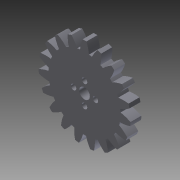
# Autodesk Inventor part: Spur Gear1
Saved by Autodesk Inventor 2013 (Build 170138000, 138)
## iProperties
Created: 2013-02-22
Part Number: Spur Gear1
Material: Steel
Document SubType Name: Modeling
Designer: Nano
Categories: <?xml version="1.0" encoding="UTF-16"?> <MemberInstance><Categories><FamilyTemplate><FamilyTemplateParameter ValueType="xs:double" Id="1" ObjectReferenceKey="da_z" ObjectType="kUserParameterObject"/><FamilyTemplateParameter ValueType="xs:double" Id="2" ObjectReferenceKey="da_b" ObjectType="kUserParameterObject"/><FamilyTemplateParameter ValueType="xs:double" Id="3" ObjectReferenceKey="da_beta" ObjectType="kUserParameterObject"/><FamilyTemplateParameter ValueType="xs:double" Id="4" ObjectReferenceKey="da_da" ObjectType="kUserParameterObject"/><FamilyTemplateParameter ValueType="xs:double" Id="5" ObjectReferenceKey="da_aw" ObjectType="kUserParameterObject"/><FamilyTemplateParameter ValueType="xs:string" Id="6" ObjectReferenceKey="EAIAABAAAAC/AAAAAAAAAIAAAAAAAAAA" ObjectType="83910656" SubObjectId="SurfaceGeometry"/></FamilyTemplate><ParamToTemplateMap><ParamToTemplate CategoryParameter="//CategoryParameter[@InternalName='046C89C9-8512-4d59-83FE-43B91F4F132A']" TemplateParameter="1"/><ParamToTemplate CategoryParameter="//CategoryParameter[@InternalName='2552DF32-E462-4b46-AEBF-C6C7768E72AC']" TemplateParameter="2"/><ParamToTemplate CategoryParameter="//CategoryParameter[@InternalName='C9EE641D-15FC-4fae-A226-E94C4372FDD7']" TemplateParameter="3"/><ParamToTemplate><ParamToTemplate CategoryParameter="//CategoryParameter[@InternalName='00B6519A-459B-49c7-AD84-2E56D39A5744']" ConstantValue="0.000000"/></ParamToTemplate><ParamToTemplate><ParamToTemplate CategoryParameter="//CategoryParameter[@InternalName='04B31F0E-C7A6-4894-AA32-9629BEFACF47']" ConstantValue="1.000000"/></ParamToTemplate><ParamToTemplate><ParamToTemplate CategoryParameter="//CategoryParameter[@InternalName='43CBEC2E-7847-49e7-A936-2F7889FCB2D9']" ConstantValue="0.250000"/></ParamToTemplate><ParamToTemplate><ParamToTemplate CategoryParameter="//CategoryParameter[@InternalName='B1EFC894-105D-4ebd-86BF-FA20ED196853']" ConstantValue="0.350000"/></ParamToTemplate><ParamToTemplate><ParamToTemplate CategoryParameter="//CategoryParameter[@InternalName='51175063-3D10-4879-93E8-6246FE8B403D']" ConstantValue="2060110000.000000"/></ParamToTemplate><ParamToTemplate><ParamToTemplate CategoryParameter="//CategoryParameter[@InternalName='A3A52E27-4454-46a9-B0BD-C932399B70AF']" ConstantValue="0.300000"/></ParamToTemplate><ParamToTemplate><ParamToTemplate CategoryParameter="//CategoryParameter[@InternalName='91B76062-C214-41d9-B1B9-14D2AB99603D']" ConstantValue="0.254000"/></ParamToTemplate><ParamToTemplate><ParamToTemplate CategoryParameter="//CategoryParameter[@InternalName='374E806E-8B8A-4dda-A9AA-1039D6500AD2']" ConstantValue="3.937008"/></ParamToTemplate><ParamToTemplate><ParamToTemplate CategoryParameter="//CategoryParameter[@InternalName='2D373A89-B862-43d6-8D0B-0CBF12AB9F6C']" ConstantValue="0.349066"/></ParamToTemplate><ParamToTemplate CategoryParameter="//CategoryParameter[@InternalName='37777632-D6A2-4fac-9D53-DB8ACD95C989']" TemplateParameter="4"/><ParamToTemplate CategoryParameter="//CategoryParameter[@InternalName='FD1017F1-B727-4f7e-9707-0F86F1FF9423']" TemplateParameter="5"/><ParamToTemplate><ParamToTemplate CategoryParameter="//CategoryParameter[@InternalName='9E1B4470-B2D3-4ff1-B813-535BB4CDF51A']" ConstantValue="3520790.000000"/></ParamToTemplate><ParamToTemplate><ParamToTemplate CategoryParameter="//CategoryParameter[@InternalName='F8452263-BFF6-458c-9FB1-07C4B99E95CD']" ConstantValue="11389170.000000"/></ParamToTemplate><ParamToTemplate><ParamToTemplate CategoryParameter="//CategoryParameter[@InternalName='3E3BB259-FD49-497f-8171-6EBC954A3479']" ConstantValue="2.000000"/></ParamToTemplate><ParamToTemplate CategoryParameter="//CategoryParameter[@InternalName='27C3BAF2-7550-4e4b-AE2C-0DB134B7D9B7']" TemplateParameter="6"/></ParamToTemplateMap><Category DisplayName="Gear" InternalName="DC85795E-93AB-48d5-8EEE-5A27447B64BD" Mnemonic="Gear"><CategoryParameter DisplayName="z" InternalName="046C89C9-8512-4d59-83FE-43B91F4F132A" Mnemonic="z"/><CategoryParameter DisplayName="b" InternalName="2552DF32-E462-4b46-AEBF-C6C7768E72AC" Mnemonic="b"/><CategoryParameter DisplayName="||b|" InternalName="C9EE641D-15FC-4fae-A226-E94C4372FDD7" Mnemonic="beta"/><CategoryParameter DisplayName="x" InternalName="00B6519A-459B-49c7-AD84-2E56D39A5744" Mnemonic="x"/><CategoryParameter DisplayName="a*" InternalName="04B31F0E-C7A6-4894-AA32-9629BEFACF47" Mnemonic="a"/><CategoryParameter DisplayName="c*" InternalName="43CBEC2E-7847-49e7-A936-2F7889FCB2D9" Mnemonic="c"/><CategoryParameter DisplayName="r|.f|*" InternalName="B1EFC894-105D-4ebd-86BF-FA20ED196853" Mnemonic="rf"/><CategoryParameter DisplayName="E" InternalName="51175063-3D10-4879-93E8-6246FE8B403D" Mnemonic="E"/><CategoryParameter DisplayName="||m|" InternalName="A3A52E27-4454-46a9-B0BD-C932399B70AF" Mnemonic="mi"/><Category DisplayName="SpurGear" InternalName="26C5A22E-A91E-4dfd-A3B3-23CCAFAE1764" Mnemonic="SpurGear"><CategoryParameter DisplayName="m" InternalName="91B76062-C214-41d9-B1B9-14D2AB99603D" Mnemonic="m"/><CategoryParameter DisplayName="P" InternalName="374E806E-8B8A-4dda-A9AA-1039D6500AD2" Mnemonic="PP"/><CategoryParameter DisplayName="||a|" InternalName="2D373A89-B862-43d6-8D0B-0CBF12AB9F6C" Mnemonic="alpha"/><CategoryParameter DisplayName="d|.a|" InternalName="37777632-D6A2-4fac-9D53-DB8ACD95C989" Mnemonic="da"/><CategoryParameter DisplayName="a|.w|" InternalName="FD1017F1-B727-4f7e-9707-0F86F1FF9423" Mnemonic="aw"/><CategoryParameter DisplayName="||s||.Flim|" InternalName="9E1B4470-B2D3-4ff1-B813-535BB4CDF51A" Mnemonic="sFlim"/><CategoryParameter DisplayName="||s||.Hlim|" InternalName="F8452263-BFF6-458c-9FB1-07C4B99E95CD" Mnemonic="sHlim"/><CategoryParameter DisplayName="type" InternalName="3E3BB259-FD49-497f-8171-6EBC954A3479" Mnemonic="type"/><CategoryParameter DisplayName="PitchDiameter" InternalName="27C3BAF2-7550-4e4b-AE2C-0DB134B7D9B7" Mnemonic="IDS_PITCHDIAM"/></Category></Category></Categories></MemberInstance>
Density: 1 g/cm^3
CustomPartVersion: 1
Author: Nano
Autodesk Inventor part; units mm, degrees
sketch "Sketch1" plane through (0, 0, 0) normal (0, 0, 1) x (1, 0, 0)
  circle A0 centre (0, 0) radius 26.67
  dimension "d0" = 53.34
  constraints: 1 centre point
  measures "d0" diameter of A0
extrude "Extrusion1" add sketch "Sketch1" along normal blind 6.35
sketch "Sketch2" plane through (0, 0, 0) normal (0, 0, -1) x (-1, 0, 0)
  circle A0 centre (0, 0) radius 26.67 projected
  circle A1 centre (0, 0) radius 24.13
  dimension "d3" = 48.26
  constraints: 1 centre point, 1 coincident
  measures "d3" diameter of A1
surface extrude "Pitch Diameter" sketch "Sketch2" against normal through all shown no curves A1
ref_plane "Work Plane1" through (0, 0, 0) normal (1, 0, 0) x (0, 1, 0)
ref_plane "Work Plane2" through (0, 0, 0) normal (0.9863613, 0.1645946, 0) x (0, 0, 1)
ref_plane "Work Plane3" through (0, 0, 3.175) normal (0, 0, -1) x (-1, 0, 0)
spur gear teeth "Spur Gear" teeth 19 pitch diameter 48.26 tip diameter 53.34 root diameter 41.91 face width 6.35 start plane through (0, 0, 0) normal (0, 0, -1) x (-1, 0, 0)
sketch "Sketch3" plane through (0, 0, 6.35) normal (0, 0, 1) x (1, 0, 0)
  arc A0 (-9.6948, 24.8455) -> (-9.2034, 18.8258) centre (10.7599, 23.4853) ccw projected
  arc A1 (-9.2034, 18.8258) -> (-10.7266, 18.0015) centre (0, 0) ccw projected
  arc A2 (-10.7266, 18.0015) -> (-15.4973, 21.7053) centre (-25.5462, 3.8374) ccw projected
  arc A3 (-15.4973, 21.7053) -> (-17.2368, 20.3515) centre (0, 0) ccw projected
  arc A4 (-17.2368, 20.3515) -> (-14.8174, 14.8174) centre (2.5512, 25.7066) ccw projected
  arc A5 (-14.8174, 14.8174) -> (-15.9904, 13.5432) centre (0, 0) ccw projected
  arc A6 (-15.9904, 13.5432) -> (-21.7053, 15.4973) centre (-25.4081, -4.6654) ccw projected
  arc A7 (-21.7053, 15.4973) -> (-22.911, 13.652) centre (0, 0) ccw projected
  arc A8 (-22.911, 13.652) -> (-18.8258, 9.2034) centre (-5.9339, 25.1421) ccw projected
  arc A9 (-18.8258, 9.2034) -> (-19.5215, 7.6173) centre (0, 0) ccw projected
  arc A10 (-19.5215, 7.6173) -> (-25.5613, 7.6099) centre (-22.5166, -12.6626) ccw projected
  arc A11 (-25.5613, 7.6099) -> (-26.1024, 5.4731) centre (0, 0) ccw projected
  arc A12 (-26.1024, 5.4731) -> (-20.7941, 2.592) centre (-13.776, 21.8531) ccw projected
  arc A13 (-20.7941, 2.592) -> (-20.9371, 0.866) centre (0, 0) ccw projected
  arc A14 (-20.9371, 0.866) -> (-26.6472, -1.1021) centre (-17.185, -19.2876) ccw projected
  arc A15 (-26.6472, -1.1021) -> (-26.4652, -3.2989) centre (0, 0) ccw projected
  arc A16 (-26.4652, -3.2989) -> (-20.509, -4.3003) centre (-20.1253, 16.196) ccw projected
  arc A17 (-20.509, -4.3003) -> (-20.0838, -5.9792) centre (0, 0) ccw projected
  arc A18 (-20.0838, -5.9792) -> (-24.8455, -9.6948) centre (-9.9912, -23.8225) ccw projected
  arc A19 (-24.8455, -9.6948) -> (-23.9601, -11.7134) centre (0, 0) ccw projected
  arc A20 (-23.9601, -11.7134) -> (-18.0015, -10.7266) centre (-24.2937, 8.7838) ccw projected
  arc A21 (-18.0015, -10.7266) -> (-17.0542, -12.1765) centre (0, 0) ccw projected
  arc A22 (-17.0542, -12.1765) -> (-20.3515, -17.2368) centre (-1.7147, -25.7759) ccw projected
  arc A23 (-20.3515, -17.2368) -> (-18.8585, -18.8585) centre (0, 0) ccw projected
  arc A24 (-18.8585, -18.8585) -> (-13.5432, -15.9904) centre (-25.8294, 0.4197) ccw projected
  arc A25 (-13.5432, -15.9904) -> (-12.1765, -17.0542) centre (0, 0) ccw projected
  arc A26 (-12.1765, -17.0542) -> (-13.652, -22.911) centre (6.7476, -24.936) ccw projected
  arc A27 (-13.652, -22.911) -> (-11.7134, -23.9601) centre (0, 0) ccw projected
  arc A28 (-11.7134, -23.9601) -> (-7.6173, -19.5215) centre (-24.5662, -7.9898) ccw projected
  arc A29 (-7.6173, -19.5215) -> (-5.9792, -20.0838) centre (0, 0) ccw projected
  arc A30 (-5.9792, -20.0838) -> (-5.4731, -26.1024) centre (14.4787, -21.394) ccw projected
  arc A31 (-5.4731, -26.1024) -> (-3.2989, -26.4652) centre (0, 0) ccw projected
  arc A32 (-3.2989, -26.4652) -> (-0.866, -20.9371) centre (-20.6408, -15.5336) ccw projected
  arc A33 (-0.866, -20.9371) -> (0.866, -20.9371) centre (0, 0) ccw projected
  arc A34 (0.866, -20.9371) -> (3.2989, -26.4652) centre (20.6408, -15.5336) ccw projected
  arc A35 (3.2989, -26.4652) -> (5.4731, -26.1024) centre (0, 0) ccw projected
  arc A36 (5.4731, -26.1024) -> (5.9792, -20.0838) centre (-14.4787, -21.394) ccw projected
  arc A37 (5.9792, -20.0838) -> (7.6173, -19.5215) centre (0, 0) ccw projected
  arc A38 (7.6173, -19.5215) -> (11.7134, -23.9601) centre (24.5662, -7.9898) ccw projected
  arc A39 (11.7134, -23.9601) -> (13.652, -22.911) centre (0, 0) ccw projected
  arc A40 (13.652, -22.911) -> (12.1765, -17.0542) centre (-6.7476, -24.936) ccw projected
  arc A41 (12.1765, -17.0542) -> (13.5432, -15.9904) centre (0, 0) ccw projected
  arc A42 (13.5432, -15.9904) -> (18.8585, -18.8585) centre (25.8294, 0.4197) ccw projected
  arc A43 (18.8585, -18.8585) -> (20.3515, -17.2368) centre (0, 0) ccw projected
  arc A44 (20.3515, -17.2368) -> (17.0542, -12.1765) centre (1.7147, -25.7759) ccw projected
  arc A45 (17.0542, -12.1765) -> (18.0015, -10.7266) centre (0, 0) ccw projected
  arc A46 (18.0015, -10.7266) -> (23.9601, -11.7134) centre (24.2937, 8.7838) ccw projected
  arc A47 (23.9601, -11.7134) -> (24.8455, -9.6948) centre (0, 0) ccw projected
  arc A48 (24.8455, -9.6948) -> (20.0838, -5.9792) centre (9.9912, -23.8225) ccw projected
  arc A49 (20.0838, -5.9792) -> (20.509, -4.3003) centre (0, 0) ccw projected
  arc A50 (20.509, -4.3003) -> (26.4652, -3.2989) centre (20.1253, 16.196) ccw projected
  arc A51 (26.4652, -3.2989) -> (26.6472, -1.1021) centre (0, 0) ccw projected
  arc A52 (26.6472, -1.1021) -> (20.9371, 0.866) centre (17.185, -19.2876) ccw projected
  arc A53 (20.9371, 0.866) -> (20.7941, 2.592) centre (0, 0) ccw projected
  arc A54 (20.7941, 2.592) -> (26.1024, 5.4731) centre (13.776, 21.8531) ccw projected
  arc A55 (26.1024, 5.4731) -> (25.5613, 7.6099) centre (0, 0) ccw projected
  arc A56 (25.5613, 7.6099) -> (19.5215, 7.6173) centre (22.5166, -12.6626) ccw projected
  arc A57 (19.5215, 7.6173) -> (18.8258, 9.2034) centre (0, 0) ccw projected
  arc A58 (18.8258, 9.2034) -> (22.911, 13.652) centre (5.9339, 25.1421) ccw projected
  arc A59 (22.911, 13.652) -> (21.7053, 15.4973) centre (0, 0) ccw projected
  arc A60 (21.7053, 15.4973) -> (15.9904, 13.5432) centre (25.4081, -4.6654) ccw projected
  arc A61 (15.9904, 13.5432) -> (14.8174, 14.8174) centre (0, 0) ccw projected
  arc A62 (14.8174, 14.8174) -> (17.2368, 20.3515) centre (-2.5512, 25.7066) ccw projected
  arc A63 (17.2368, 20.3515) -> (15.4973, 21.7053) centre (0, 0) ccw projected
  arc A64 (15.4973, 21.7053) -> (10.7266, 18.0015) centre (25.5462, 3.8374) ccw projected
  arc A65 (10.7266, 18.0015) -> (9.2034, 18.8258) centre (0, 0) ccw projected
  arc A66 (9.2034, 18.8258) -> (9.6948, 24.8455) centre (-10.7599, 23.4853) ccw projected
  arc A67 (9.6948, 24.8455) -> (7.6099, 25.5613) centre (0, 0) ccw projected
  arc A68 (7.6099, 25.5613) -> (4.3003, 20.509) centre (22.9161, 11.9243) ccw projected
  arc A69 (4.3003, 20.509) -> (2.592, 20.7941) centre (0, 0) ccw projected
  arc A70 (2.592, 20.7941) -> (1.1021, 26.6472) centre (-17.8026, 18.7191) ccw projected
  arc A71 (1.1021, 26.6472) -> (-1.1021, 26.6472) centre (0, 0) ccw projected
  arc A72 (-1.1021, 26.6472) -> (-2.592, 20.7941) centre (17.8026, 18.7191) ccw projected
  arc A73 (-2.592, 20.7941) -> (-4.3003, 20.509) centre (0, 0) ccw projected
  arc A74 (-4.3003, 20.509) -> (-7.6099, 25.5613) centre (-22.9161, 11.9243) ccw projected
  arc A75 (-7.6099, 25.5613) -> (-9.6948, 24.8455) centre (0, 0) ccw projected
hole "Hole1" at (0, 0, 6.35) direction (0, 0, -1) diameter 6.1722 end through all
sketch "Sketch4" plane through (0, 0, 6.35) normal (0, 0, 1) x (1, 0, 0)
  circle A0 centre (0, 0) radius 3.0861 projected
  point P0 (-6.35, 0)
  dimension "d37" = 6.35
  measures "d37" distance of A0.centre point (-6.35, 0)
hole "Hole2" at (-6.35, 0, 6.35) direction (0, 0, -1) diameter 3.175 end through all
pattern_circular "Circular Pattern1" count 4 over 360 about axis through (0, 0, -69.1746) along (0, 0, 1) of "Hole2"
equation "\"d0\" = da_da"
equation "\"d1\" = da_b"
equation "\"d3\" = da_dw"
equation "\"d15\" = da_aw"
equation "\"d19\" = da_aw"
equation "\"da_da\" = 53.34"
equation "\"da_b\" = 6.35"
equation "\"da_dw\" = 48.26"
equation "\"da_aw\" = 195.58"
body "Solid1"
body "Srf1"
